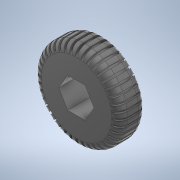
# Autodesk Inventor part: standoffAdapter
Saved by Autodesk Inventor 2020.4 (Build 244396000, 396)
## iProperties
Created: 2019-10-04
Part Number: standoffAdapter
Material: Generic
Document SubType Name: Modeling
Designer: Acer
Density: 1 g/cm^3
Appearance: Default
Author: Acer
Autodesk Inventor part; units mm, degrees
ref_plane "YZ Plane" through (0, 0, 0) normal (1, 0, 0) x (0, 1, 0)
ref_plane "XZ Plane" through (0, 0, 0) normal (0, 1, 0) x (-1, 0, 0)
ref_plane "XY Plane" through (0, 0, 0) normal (0, 0, 1) x (1, 0, 0)
sketch "Sketch1" plane through (0, 0, 0) normal (0, 0, 1) x (1, 0, 0)
  line L0 (-1.6166, -2.8) -> (-3.2332, 0)
  line L1 (-3.2332, 0) -> (-1.6166, 2.8)
  line L2 (-1.6166, 2.8) -> (1.6166, 2.8)
  line L3 (1.6166, 2.8) -> (3.2332, 0)
  line L4 (3.2332, 0) -> (1.6166, -2.8)
  line L5 (1.6166, -2.8) -> (-1.6166, -2.8)
  circle A0 centre (0, 0) radius 8
  dimension "d1" = 5.6
  dimension "d2" = 16
  constraints: 12 end point, 2 coincident, 1 centre point, 1 horizontal, 13 other
  measures "d1" distance between parallel lines of L2 L5
  measures "d2" diameter of A0
extrude "Extrusion1" add sketch "Sketch1" along normal blind 5
fillet "Fillet1" radius 1.5 2 edges at (-8, 0, 5) (-8, 0, 0)
sketch "Sketch2" plane through (0, 0, 0) normal (0, 1, 0) x (-1, 0, 0)
  line L0 (-8, 0) -> (-8, 5) projected
  line L1 (8, 5) -> (-8, 5) projected
  line L2 (8, 0) -> (-8, 0) projected
  arc A0 (-6.5, 5) -> (-6.5, 0) centre (-4.75, 2.5) ccw
  line L3 (-6.5, 5) -> (-6.5, 0) construction
  line L4 (-6.5, 5) -> (-1.5, 5) construction
  point P0 (0, 0)
  dimension "d5" = 90
  dimension "d6" = 6.5
  dimension "d7" = 3.25
  constraints: 4 end point, 2 point on circle, 2 point on line, 1 centre point, 1 horizontal, 1 perpendicular
  measures "d5" angle of L3 L4
  measures "d6" distance of point (0, 0) L3.end
  measures "d7" distance from line of L0 A0.centre
extrude "Extrusion2" cut sketch "Sketch2" against normal mid plane 0.4
pattern_circular "Circular Pattern1" count 40 over 360 about axis through (0, 0, -10) along (0, 0, 1) of "Extrusion2"
body "Solid1"
